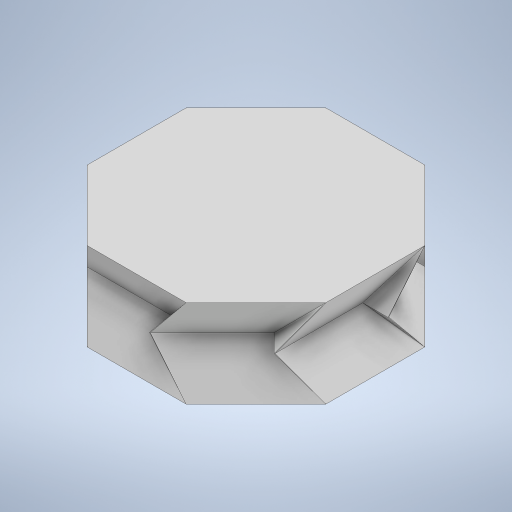
# Autodesk Inventor part: 팔각형 OV-PAM 층 한개
Saved by Autodesk Inventor 2024 (Build 280153000, 153)
## iProperties
Created: 2023-06-16
Part Number: 팔각형 OV-PAM 층 한개
Material: 일반
Document SubType Name: Modeling
Designer: jsw
Density: 1 g/cm^3
Appearance: 기본값
Author: jsw
Autodesk Inventor part; units mm, degrees
ref_plane "YZ Plane" through (0, 0, 0) normal (1, 0, 0) x (0, 1, 0)
ref_plane "XZ Plane" through (0, 0, 0) normal (0, 1, 0) x (-1, 0, 0)
sketch "스케치1" plane through (0, 0, 0) normal (0, 1, 0) x (-1, 0, 0)
  line L0 (-31.9919, 13.2515) -> (-13.2515, 31.9919)
  line L1 (-13.2515, 31.9919) -> (13.2515, 31.9919)
  line L2 (13.2515, 31.9919) -> (31.9919, 13.2515)
  line L3 (31.9919, 13.2515) -> (31.9919, -13.2515)
  line L4 (31.9919, -13.2515) -> (13.2515, -31.9919)
  line L5 (13.2515, -31.9919) -> (-13.2515, -31.9919)
  line L6 (-13.2515, -31.9919) -> (-31.9919, -13.2515)
  line L7 (-31.9919, -13.2515) -> (-31.9919, 13.2515)
  line L8 (-13.5, 32.5919) -> (13.5, 32.5919)
  line L9 (13.5, 32.5919) -> (32.5919, 13.5)
  line L10 (32.5919, 13.5) -> (32.5919, -13.5)
  line L11 (32.5919, -13.5) -> (13.5, -32.5919)
  line L12 (13.5, -32.5919) -> (-13.5, -32.5919)
  line L13 (-13.5, -32.5919) -> (-32.5919, -13.5)
  line L14 (-32.5919, -13.5) -> (-32.5919, 13.5)
  line L15 (-32.5919, 13.5) -> (-13.5, 32.5919)
  point P0 (0, 0)
  point P1 (0, 0)
  point P2 (0, 0)
  dimension "d2" = 0.6
  dimension "d53" = 27
  constraints: 32 end point, 2 coincident, 2 horizontal, 34 other
  measures "d2" distance between parallel lines of L10 L3
  measures "d53" distance of L9.end L10.end
extrude "돌출2" add sketch "스케치1" along normal blind 12 contours L0 L1 L2 L3 L4 L5 L6 L7 | L8 L9 L10 L11 L12 L13 L14 L15
ref_plane "작업 평면2" through (32.5919, 0, 13.5) normal (-0.8660254, -0.5, 0) x (0, 0, -1)
sketch "스케치3" plane through (32.5919, 0, 13.5) normal (1, 0, 0) x (0, 0, -1)
  line L0 (0, 0) -> (0, 12) projected
  line L1 (0, 12) -> (27, 12) projected
  line L2 (0, 0) -> (27, 0)
  line L3 (27, 0) -> (27, 12)
  line L4 (27, 12) -> (0, 12)
  line L5 (0, 12) -> (0, 0)
  line L6 (0, 12) -> (-7.3047, 12)
  line L7 (-19.0919, 12) -> (0, 12) projected
  line L8 (0, 0) -> (-7.3047, 12)
  line L9 (27, 12) -> (13.5, 12)
  line L10 (17, 12) -> (27, 0)
  point P0 (13.5, 0)
  point P1 (17, 12)
  dimension "d17" = 121.33
  dimension "d49" = 3.5
  constraints: 16 end point, 5 midpoint, 2 parallel, 2 point on line, 1 horizontal, 1 perpendicular
  measures "d17" angle of L8 L2
  measures "d49" distance of point (13.5, 12) L10.start
extrude "돌출4" cut sketch "스케치3" against normal up to surface contours L8 L6 L0 | L0 L1 L10 L2 surface through (32.5919, 0, 13.5) normal (-0.8660254, -0.5, 0)
pattern_circular "원형 패턴1" count 8 over 360 about axis through (0, -10, 0) along (0, 1, 0) of "돌출4"
mirror "미러5" about plane through (0, 12, 0) normal (0, 1, 0) of "돌출2", "돌출4", "원형 패턴1"
